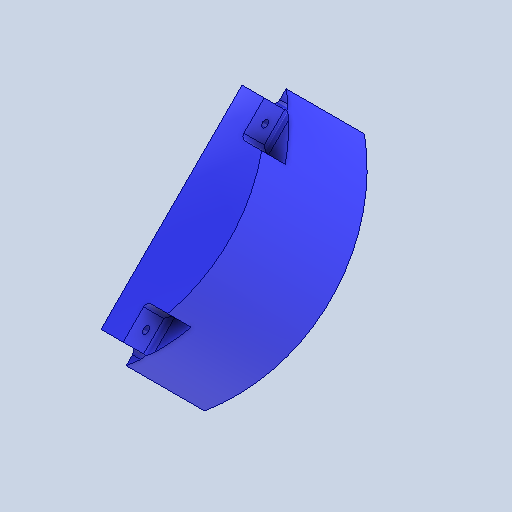
# Autodesk Inventor part: base_weel-v2-3DP-1
Saved by Autodesk Inventor 2025.2 (Build 292293000, 293)
## iProperties
Created: 2025-04-01
Part Number: base_weel-v2-3DP-1
Material: ABS プラスチック
Document SubType Name: Modeling
Designer: haruy
Density: 1.06 g/cm^3
Appearance: 青 - 壁塗料 - 光沢
Author: haruy
Autodesk Inventor part; units mm, degrees
ref_plane "YZ Plane" through (0, 0, 0) normal (1, 0, 0) x (0, 1, 0)
ref_plane "XZ Plane" through (0, 0, 0) normal (0, 1, 0) x (-1, 0, 0)
ref_plane "XY Plane" through (0, 0, 0) normal (0, 0, 1) x (1, 0, 0)
derived "base_weel-v2-Sketch-Base.ipt"
sketch "スケッチ1" plane through (0, 0, 0) normal (1, 0, 0) x (0, 1, 0)
  line L0 (-315, 315) -> (315, 315)
  line L1 (315, 315) -> (315, -315)
  line L2 (315, -315) -> (-315, -315)
  line L3 (-315, -315) -> (-315, 315)
  line L4 (-315, 315) -> (315, -315) construction
  line L5 (315, 315) -> (-315, -315) construction
  line L6 (-295, 218) -> (-295, -202)
  line L7 (-295, -202) -> (-315, -202)
  line L8 (-315, -202) -> (-315, 210)
  line L9 (242, 315) -> (-242, 315)
  line L10 (-242, 315) -> (-242, 295)
  line L11 (-242, 295) -> (242, 295)
  line L12 (242, 295) -> (242, 315)
  line L13 (-295, 218) -> (-295, 315)
  line L14 (0, 0) -> (-956.597305, 0)
  circle A0 centre (0, 0) radius 400
  line L15 (-330, 25) -> (-380, 25)
  line L16 (-380, 25) -> (-380, -25)
  line L17 (-380, -25) -> (-330, -25)
  line L18 (-330, -25) -> (-330, 25)
  line L19 (0, 0) -> (0, -630.91786)
  line L20 (-315, 40) -> (-395, 40)
  line L21 (-395, 40) -> (-395, 30)
  line L22 (-395, 30) -> (-315, 30)
  line L23 (-315, 30) -> (-315, 40)
  line L24 (-395, 30) -> (-385, 30)
  line L25 (-385, 30) -> (-385, 0)
  line L26 (-385, 0) -> (-395, 0)
  line L27 (-395, 0) -> (-395, 30)
  line L28 (295, 202) -> (315, 202)
  line L29 (315, 202) -> (315, -202)
  line L30 (315, -202) -> (295, -202)
  line L31 (295, -202) -> (295, 202)
  line L32 (-222.218254, -315) -> (242, -315)
  line L33 (242, -315) -> (242, -295)
  line L34 (242, -295) -> (-242, -295)
  line L35 (315, 315) -> (0, 0)
  line L36 (315, 125) -> (315, 145)
  circle A1 centre (548.476864, 0) radius 122.5
  circle A2 centre (179.690493, 0) radius 600
  circle A3 centre (548.476864, 0) radius 200
  circle A4 centre (0, 0) radius 10
  arc A5 (0, 150) -> (0, -150) centre (0, 0) ccw
  arc A6 (0, 140) -> (0, -140) centre (0, 0) ccw
  line L37 (-146.327154, 32.990361) -> (-136.572011, 30.791004)
  line L38 (-137.581214, 37.681687) -> (-140.440379, 25)
  line L39 (-140.440379, 25) -> (-145.317951, 26.099679)
  line L40 (-145.317951, 26.099679) -> (-142.458786, 38.781365)
  line L41 (-142.458786, 38.781365) -> (-137.581214, 37.681687)
  arc A7 (-29.130183, 142.04377) -> (-29.130183, -142.04377) centre (0, 0) ccw
  circle A8 centre (-151.490382, 39.279944) radius 6.5
  circle A9 centre (-129.040116, 34.218393) radius 6.5 construction
  circle A10 centre (-129.040116, 34.218393) radius 1.5 construction
  circle A11 centre (-151.490382, 39.279944) radius 1.5
  line L42 (-30.166794, 22.5) -> (-174.136226, 22.5)
  line L43 (-174.136226, 22.5) -> (-174.136226, 7.5)
  line L44 (-174.136226, 7.5) -> (-30.166794, 7.5)
  line L45 (-30.166794, 7.5) -> (-30.166794, 22.5)
  circle A12 centre (-129.040116, -34.218393) radius 6.5 construction
  circle A13 centre (-129.040116, -34.218393) radius 1.5 construction
  line L46 (-142.458786, -38.781365) -> (-137.581214, -37.681687)
  line L47 (-145.317951, -26.099679) -> (-142.458786, -38.781365)
  line L48 (-137.581214, -37.681687) -> (-140.440379, -25)
  line L49 (-140.440379, -25) -> (-145.317951, -26.099679)
  circle A14 centre (-151.490382, -39.279944) radius 6.5
  circle A15 centre (-151.490382, -39.279944) radius 1.5
  line L50 (-146.327154, -32.990361) -> (-136.572011, -30.791004)
  line L51 (-30.166794, -22.5) -> (-174.136226, -22.5)
  line L52 (-174.136226, -7.5) -> (-30.166794, -7.5)
  line L53 (-30.166794, -7.5) -> (-30.166794, -22.5)
  line L54 (-174.136226, -22.5) -> (-174.136226, -7.5)
  line L55 (-151.490382, 39.279944) -> (-129.040116, 34.218393) construction
  line L56 (-129.040116, 34.218393) -> (-129.589956, 31.779607) construction
  line L57 (-129.589956, 31.779607) -> (-152.040222, 36.841158) construction
  line L58 (-152.040222, 36.841158) -> (-151.490382, 39.279944) construction
  line L59 (-129.040116, 34.218393) -> (-151.490382, 39.279944) construction
  line L60 (-151.490382, 39.279944) -> (-150.940543, 41.71873) construction
  line L61 (-150.940543, 41.71873) -> (-128.490277, 36.657179) construction
  line L62 (-128.490277, 36.657179) -> (-129.040116, 34.218393) construction
  line L63 (-128.490277, 36.657179) -> (-129.589956, 31.779607) construction
  line L64 (-129.589956, 31.779607) -> (-117.883783, 29.140378) construction
  line L65 (-117.883783, 29.140378) -> (-116.784104, 34.01795) construction
  line L66 (-116.784104, 34.01795) -> (-128.490277, 36.657179) construction
  line L67 (-150.940543, 41.71873) -> (-152.040222, 36.841158) construction
  line L68 (-152.040222, 36.841158) -> (-163.746394, 39.480387) construction
  line L69 (-163.746394, 39.480387) -> (-162.646715, 44.357959) construction
  line L70 (-162.646715, 44.357959) -> (-150.940543, 41.71873) construction
  line L71 (-155.268276, 45.257195) -> (-128.941244, 39.321603)
  line L72 (-128.941244, 39.321603) -> (-132.24028, 24.688887)
  line L73 (-132.24028, 24.688887) -> (-158.567312, 30.624479)
  line L74 (-158.567312, 30.624479) -> (-155.268276, 45.257195)
  line L75 (-128.941244, -39.321603) -> (-132.24028, -24.688887)
  line L76 (-155.268276, -45.257195) -> (-128.941244, -39.321603)
  line L77 (-132.24028, -24.688887) -> (-158.567312, -30.624479)
  line L78 (-158.567312, -30.624479) -> (-155.268276, -45.257195)
  arc A16 (-132.24028, 24.688887) -> (-132.24028, -24.688887) centre (0, 0) ccw
  arc A17 (-158.567312, 30.624479) -> (-158.567312, -30.624479) centre (0, 0) ccw
  circle A18 centre (-152.5, 15) radius 1.25
  line L79 (-145, 0) -> (-145, 74.738194)
  circle A19 centre (-137.5, 15) radius 1.25
  circle A20 centre (-137.5, -15) radius 1.25
  circle A21 centre (-152.5, -15) radius 1.25
  line L80 (0, 0) -> (0, 140)
  line L81 (0, 0) -> (-47.88282, 131.556967)
  line L82 (0, 140) -> (0, 150)
  line L83 (-137.584562, 25.893789) -> (-134.285526, 40.526504)
  line L84 (-137.584562, -25.893789) -> (-134.285526, -40.526504)
  circle A22 centre (0, 0) radius 20
  line L85 (295, 45) -> (-295, 45)
  line L86 (-295, 45) -> (-295, 25)
  line L87 (-295, 25) -> (295, 25)
  line L88 (295, 25) -> (295, 45)
  line L89 (-40, 295) -> (-50, 295)
  line L90 (-50, 295) -> (-50, 45)
  line L91 (-50, 45) -> (-40, 45)
  line L92 (-40, 45) -> (-40, 295)
  line L93 (-50, -295) -> (-50, -45)
  line L94 (-40, -45) -> (-40, -295)
  line L95 (295, -45) -> (-295, -45)
  line L96 (-295, -25) -> (295, -25)
  line L97 (-40, 45) -> (-40, -45)
  line L98 (40, 45) -> (40, -45)
  circle A23 centre (20, 35) radius 1.5
  circle A24 centre (-20, 35) radius 1.5
  circle A25 centre (-20, -35) radius 1.5
  circle A26 centre (20, -35) radius 1.5
  circle A27 centre (-45, 125) radius 1.5
  circle A28 centre (-45, 125) radius 5
  circle A29 centre (-130, 35) radius 5
  circle A30 centre (-130, 35) radius 1.5
  line L99 (-40, 134.164079) -> (-40, 125)
  line L100 (-50, 125) -> (-50, 130.766968)
  line L101 (-137.749773, 25) -> (-127.580079, 30.624616)
  line L102 (-132.570736, 45) -> (-126.365969, 38.434213)
  line L103 (-40, -134.164079) -> (-40, -125)
  circle A31 centre (-45, -125) radius 5
  circle A32 centre (-45, -125) radius 1.5
  line L104 (-50, -125) -> (-50, -130.766968)
  line L105 (-132.570736, -45) -> (-126.365969, -38.434213)
  circle A33 centre (-130, -35) radius 5
  circle A34 centre (-130, -35) radius 1.5
  line L106 (-137.749773, -25) -> (-127.580079, -30.624616)
  line L107 (-242, -295) -> (-242, -315)
  line L108 (242, 315) -> (222, 315)
  line L109 (222, 315) -> (222, 295)
  line L110 (222, 295) -> (242, 295)
  line L111 (242, 295) -> (242, 315)
  line L112 (242, -315) -> (222, -315)
  line L113 (222, -315) -> (222, -295)
  line L114 (222, -295) -> (242, -295)
  line L115 (242, -295) -> (242, -315)
  line L116 (197, 295) -> (295, 197)
  line L117 (295, 197) -> (284.393398, 186.393398)
  line L118 (284.393398, 186.393398) -> (186.393398, 284.393398)
  line L119 (186.393398, 284.393398) -> (197, 295)
  line L120 (197, 295) -> (197, 315)
  line L121 (197.916739, 294.083261) -> (187.310137, 283.476659)
  line L122 (198.270292, 272.516504) -> (272.516504, 198.270292)
  line L123 (272.516504, 198.270292) -> (231.504311, 157.258099)
  line L124 (231.504311, 157.258099) -> (157.258099, 231.504311)
  line L125 (157.258099, 231.504311) -> (198.270292, 272.516504)
  line L126 (290.901281, 201.098719) -> (280.294679, 190.492118)
  line L127 (93.76241, 295) -> (295, 93.76241)
  line L128 (295, 93.76241) -> (284.393398, 83.155808)
  line L129 (284.393398, 83.155808) -> (83.155808, 284.393398)
  line L130 (214.180195, 277.819805) -> (203.573593, 267.213203)
  line L131 (277.819805, 214.180195) -> (267.213203, 203.573593)
  circle A35 centre (199.684506, 281.708892) radius 1.5
  circle A36 centre (213.826641, 267.566757) radius 1.6
  line L132 (186.393398, 284.393398) -> (175.786797, 295)
  circle A37 centre (187, 305) radius 1.5
  circle A38 centre (177, 305) radius 1.5
  line L133 (172, 315) -> (172, 295)
  line L134 (93.76241, 295) -> (93.76241, 295)
  line L135 (93.76241, 295) -> (93.76241, 315)
  line L136 (83.155808, 284.393398) -> (72.549207, 295)
  line L137 (68.76241, 315) -> (68.76241, 295)
  line L138 (284.393398, 186.393398) -> (295, 175.786797)
  line L139 (295, 197) -> (315, 197)
  line L140 (295, 93.76241) -> (295, 93.76241)
  line L141 (284.393398, 83.155808) -> (295, 72.549207)
  line L142 (-197, 295) -> (-197, 315)
  line L143 (-172, 315) -> (-172, 295)
  line L144 (-93.76241, 295) -> (-93.76241, 315)
  line L145 (-68.76241, 315) -> (-68.76241, 295)
  line L146 (-83.155808, 284.393398) -> (-72.549207, 295)
  line L147 (-93.76241, 295) -> (-295, 93.76241)
  line L148 (-83.155808, 284.393398) -> (-93.76241, 295)
  line L149 (-284.393398, 83.155808) -> (-83.155808, 284.393398)
  line L150 (-295, 93.76241) -> (-284.393398, 83.155808)
  line L151 (-284.393398, 83.155808) -> (-295, 72.549207)
  line L152 (-272.516504, 198.270292) -> (-231.504311, 157.258099)
  line L153 (-157.258099, 231.504311) -> (-198.270292, 272.516504)
  line L154 (-284.393398, 186.393398) -> (-186.393398, 284.393398)
  line L155 (-186.393398, 284.393398) -> (-175.786797, 295)
  line L156 (-197, 295) -> (-295, 197)
  line L157 (-197.916739, 294.083261) -> (-187.310137, 283.476659)
  line L158 (-214.180195, 277.819805) -> (-203.573593, 267.213203)
  line L159 (-290.901281, 201.098719) -> (-280.294679, 190.492118)
  line L160 (-284.393398, 186.393398) -> (-295, 175.786797)
  line L161 (-295, 197) -> (-315, 197)
  line L162 (-93.76241, -295) -> (-295, -93.76241)
  line L163 (-284.393398, -83.155808) -> (-83.155808, -284.393398)
  line L164 (-295, -93.76241) -> (-284.393398, -83.155808)
  line L165 (-197, -295) -> (-295, -197)
  line L166 (-284.393398, -186.393398) -> (-186.393398, -284.393398)
  line L167 (-290.901281, -201.098719) -> (-280.294679, -190.492118)
  line L168 (-214.180195, -277.819805) -> (-203.573593, -267.213203)
  line L169 (-197.916739, -294.083261) -> (-187.310137, -283.476659)
  line L170 (-83.155808, -284.393398) -> (-93.76241, -295)
  line L171 (284.393398, -83.155808) -> (83.155808, -284.393398)
  line L172 (83.155808, -284.393398) -> (93.76241, -295)
  line L173 (93.76241, -295) -> (295, -93.76241)
  line L174 (284.393398, -186.393398) -> (186.393398, -284.393398)
  line L175 (197.916739, -294.083261) -> (187.310137, -283.476659)
  line L176 (197, -295) -> (295, -197)
  line L177 (290.901281, -201.098719) -> (280.294679, -190.492118)
  line L178 (295, -93.76241) -> (284.393398, -83.155808)
  line L179 (242, 295) -> (222, 295)
  arc A39 (0, 86) -> (0, -86) centre (0, 0) ccw construction
  circle A40 centre (-90.866661, 48.5) radius 21
  circle A41 centre (0, 0) radius 124
  circle A42 centre (-90.866661, 48.5) radius 17
  arc A43 (40.495146, 75.869251) -> (0, 86) centre (0, 0) ccw construction
  line L180 (-40, 45) -> (-50, 45)
  line L181 (-50, 45) -> (-50, -45)
  line L182 (-50, -45) -> (-40, -45)
  line L183 (-40, -45) -> (-40, 45)
  line L184 (-40, 295) -> (-50, 295)
  line L185 (-50, 295) -> (-50, 315)
  line L186 (-50, 315) -> (-40, 315)
  line L187 (-40, 315) -> (-40, 295)
  line L188 (-40, -295) -> (-50, -295)
  line L189 (-50, -295) -> (-50, -315)
  line L190 (-50, -315) -> (-40, -315)
  line L191 (-40, -315) -> (-40, -295)
  line L192 (40, -315) -> (40, -295)
  line L193 (50, -295) -> (50, -315)
  line L194 (50, -295) -> (50, -45)
  line L195 (40, -45) -> (40, -295)
  line L196 (40, -45) -> (40, 45)
  line L197 (50, 45) -> (50, -45)
  line L198 (40, 45) -> (40, 295)
  line L199 (50, 295) -> (50, 45)
  line L200 (40, 315) -> (40, 295)
  line L201 (50, 295) -> (50, 315)
  line L202 (-40.409176, 123.019006) -> (-35, 135.554417)
  line L203 (-48.741703, 121.683426) -> (-55, 128.743932)
  line L204 (-40.409176, -123.019006) -> (-35, -135.554417)
  line L205 (-48.741703, -121.683426) -> (-55, -128.743932)
  arc A44 (40.495146, 75.869251) -> (-40.495146, -75.869251) centre (0, 0) ccw
  circle A45 centre (0, 0) radius 86 construction
  circle A46 centre (0, 0) radius 78.5
  circle A47 centre (-45, 58) radius 1.5
  circle A48 centre (-45, 58) radius 5
  circle A49 centre (45, 58) radius 5
  circle A50 centre (45, 58) radius 1.5
  line L206 (46.554886, 53.247913) -> (55, 56.01116)
  line L207 (40.325005, 56.226748) -> (35, 70.265568)
  line L208 (50, 60.516527) -> (50, 69.971423)
  arc A51 (50, 69.971423) -> (40.495146, 75.869251) centre (0, 0) ccw
  line L209 (-40.325005, 56.226748) -> (-35, 70.265568)
  line L210 (-46.554886, 53.247913) -> (-55, 56.01116)
  line L211 (-40.325005, -56.226748) -> (-35, -70.265568) construction
  circle A52 centre (-45, -58) radius 5
  line L212 (-46.554886, -53.247913) -> (-55, -56.01116)
  circle A53 centre (-45, -58) radius 1.5
  line L213 (-40, -67.54443) -> (-40, -76.131465)
  arc A54 (-40.525953, -75.852799) -> (-40, -76.131465) centre (0, 0) ccw
  line L214 (-40, -76.131465) -> (-40, -58)
  line L215 (222.665476, 269.334524) -> (212.058875, 258.727922)
  line L216 (269.334524, 222.665476) -> (258.727922, 212.058875)
  circle A55 centre (267.566757, 213.826641) radius 1.6
  circle A56 centre (281.708892, 199.684506) radius 1.5
  line L217 (294.083261, 197.916739) -> (283.476659, 187.310137)
  line L218 (315, 172) -> (295, 172)
  circle A57 centre (305, 177) radius 1.5
  circle A58 centre (305, 187) radius 1.5
  line L219 (295, 197) -> (315, 197)
  circle A59 centre (83.76241, 305) radius 1.5
  circle A60 centre (73.76241, 305) radius 1.5
  line L220 (197.916739, 294.083261) -> (94.679149, 294.083261)
  line L221 (187.310137, 283.476659) -> (84.072547, 283.476659)
  line L222 (94.679149, 294.083261) -> (84.072547, 283.476659)
  circle A61 centre (96.446916, 281.708892) radius 1.5
  circle A62 centre (110.589051, 267.566757) radius 1.5
  line L223 (119.427886, 269.334524) -> (108.821284, 258.727922)
  line L224 (295, 93.76241) -> (315, 93.76241)
  line L225 (315, 68.76241) -> (295, 68.76241)
  circle A63 centre (305, 73.76241) radius 1.5
  circle A64 centre (305, 83.76241) radius 1.5
  line L226 (294.083261, 94.679149) -> (283.476659, 84.072547)
  circle A65 centre (281.708892, 96.446916) radius 1.5
  circle A66 centre (267.566757, 110.589051) radius 1.5
  line L227 (269.334524, 119.427886) -> (258.727922, 108.821284)
  line L228 (-197, 295) -> (-197, 315)
  line L229 (-172, 315) -> (-172, 295)
  circle A67 centre (-177, 305) radius 1.5
  circle A68 centre (-187, 305) radius 1.5
  line L230 (-197.916739, 294.083261) -> (-187.310137, 283.476659)
  circle A69 centre (-199.684506, 281.708892) radius 1.5
  line L231 (-214.180195, 277.819805) -> (-203.573593, 267.213203)
  circle A70 centre (-213.826641, 267.566757) radius 1.6
  line L232 (-222.665476, 269.334524) -> (-212.058875, 258.727922)
  circle A71 centre (-267.566757, 213.826641) radius 1.6
  line L233 (-269.334524, 222.665476) -> (-258.727922, 212.058875)
  circle A72 centre (-281.708892, 199.684506) radius 1.5
  line L234 (-294.083261, 197.916739) -> (-283.476659, 187.310137)
  line L235 (-295, 197) -> (-315, 197)
  circle A73 centre (-305, 187) radius 1.5
  circle A74 centre (-305, 177) radius 1.5
  line L236 (-315, 172) -> (-295, 172)
  line L237 (-295, 93.76241) -> (-315, 93.76241)
  line L238 (-315, 68.76241) -> (-295, 68.76241)
  circle A75 centre (-305, 73.76241) radius 1.5
  circle A76 centre (-305, 83.76241) radius 1.5
  line L239 (-294.083261, 94.679149) -> (-283.476659, 84.072547)
  circle A77 centre (-281.708892, 96.446916) radius 1.5
  circle A78 centre (-267.566757, 110.589051) radius 1.5
  line L240 (-269.334524, 119.427886) -> (-258.727922, 108.821284)
  line L241 (-119.427886, 269.334524) -> (-108.821284, 258.727922)
  circle A79 centre (-110.589051, 267.566757) radius 1.5
  circle A80 centre (-96.446916, 281.708892) radius 1.5
  line L242 (-94.679149, 294.083261) -> (-84.072547, 283.476659)
  line L243 (-93.76241, 295) -> (-93.76241, 315)
  line L244 (-68.76241, 315) -> (-68.76241, 295)
  circle A81 centre (-73.76241, 305) radius 1.5
  circle A82 centre (-83.76241, 305) radius 1.5
  line L245 (-295, -197) -> (-315, -197)
  circle A83 centre (-305, -187) radius 1.5
  circle A84 centre (-305, -177) radius 1.5
  line L246 (-315, -172) -> (-295, -172)
  line L247 (-294.083261, -197.916739) -> (-283.476659, -187.310137)
  circle A85 centre (-281.708892, -199.684506) radius 1.5
  circle A86 centre (-267.566757, -213.826641) radius 1.6
  line L248 (-269.334524, -222.665476) -> (-258.727922, -212.058875)
  line L249 (-222.665476, -269.334524) -> (-212.058875, -258.727922)
  circle A87 centre (-213.826641, -267.566757) radius 1.6
  circle A88 centre (-199.684506, -281.708892) radius 1.5
  line L250 (-197.916739, -294.083261) -> (-187.310137, -283.476659)
  line L251 (-197, -295) -> (-197, -315)
  circle A89 centre (-187, -305) radius 1.5
  circle A90 centre (-177, -305) radius 1.5
  line L252 (-172, -315) -> (-172, -295)
  line L253 (-295, -93.76241) -> (-315, -93.76241)
  circle A91 centre (-305, -83.76241) radius 1.5
  circle A92 centre (-305, -73.76241) radius 1.5
  line L254 (-315, -68.76241) -> (-295, -68.76241)
  line L255 (-294.083261, -94.679149) -> (-283.476659, -84.072547)
  circle A93 centre (-281.708892, -96.446916) radius 1.5
  circle A94 centre (-267.566757, -110.589051) radius 1.5
  line L256 (-269.334524, -119.427886) -> (-258.727922, -108.821284)
  line L257 (-119.427886, -269.334524) -> (-108.821284, -258.727922)
  circle A95 centre (-110.589051, -267.566757) radius 1.5
  circle A96 centre (-96.446916, -281.708892) radius 1.5
  line L258 (-94.679149, -294.083261) -> (-84.072547, -283.476659)
  line L259 (-93.76241, -295) -> (-93.76241, -315)
  circle A97 centre (-83.76241, -305) radius 1.5
  circle A98 centre (-73.76241, -305) radius 1.5
  line L260 (-68.76241, -315) -> (-68.76241, -295)
  line L261 (68.76241, -315) -> (68.76241, -295)
  circle A99 centre (73.76241, -305) radius 1.5
  circle A100 centre (83.76241, -305) radius 1.5
  line L262 (93.76241, -295) -> (93.76241, -315)
  line L263 (94.679149, -294.083261) -> (84.072547, -283.476659)
  circle A101 centre (96.446916, -281.708892) radius 1.5
  circle A102 centre (110.589051, -267.566757) radius 1.5
  line L264 (119.427886, -269.334524) -> (108.821284, -258.727922)
  line L265 (172, -315) -> (172, -295)
  circle A103 centre (177, -305) radius 1.5
  circle A104 centre (187, -305) radius 1.5
  line L266 (197, -295) -> (197, -315)
  line L267 (197.916739, -294.083261) -> (187.310137, -283.476659)
  circle A105 centre (199.684506, -281.708892) radius 1.5
  circle A106 centre (213.826641, -267.566757) radius 1.6
  line L268 (222.665476, -269.334524) -> (212.058875, -258.727922)
  line L269 (269.334524, -222.665476) -> (258.727922, -212.058875)
  circle A107 centre (267.566757, -213.826641) radius 1.6
  circle A108 centre (281.708892, -199.684506) radius 1.5
  line L270 (294.083261, -197.916739) -> (283.476659, -187.310137)
  line L271 (295, -197) -> (315, -197)
  circle A109 centre (305, -187) radius 1.5
  circle A110 centre (305, -177) radius 1.5
  line L272 (315, -172) -> (295, -172)
  line L273 (295, -93.76241) -> (315, -93.76241)
  circle A111 centre (305, -83.76241) radius 1.5
  circle A112 centre (305, -73.76241) radius 1.5
  line L274 (315, -68.76241) -> (295, -68.76241)
  line L275 (294.083261, -94.679149) -> (283.476659, -84.072547)
  circle A113 centre (281.708892, -96.446916) radius 1.5
  line L276 (269.334524, -119.427886) -> (258.727922, -108.821284)
  circle A114 centre (267.566757, -110.589051) radius 1.5
  line L277 (-295, 202) -> (-315, 202)
  line L278 (265, 45) -> (265, 25)
  circle A115 centre (275, 35) radius 1.5
  circle A116 centre (285, 35) radius 1.5
  circle A117 centre (305, 35) radius 1.5
  circle A118 centre (305, 25) radius 1.5
  line L279 (295, 25) -> (315, 25)
  line L280 (265, -45) -> (265, -25)
  circle A119 centre (275, -35) radius 1.5
  circle A120 centre (285, -35) radius 1.5
  circle A121 centre (305, -35) radius 1.5
  circle A122 centre (305, -25) radius 1.5
  circle A123 centre (-305, -25) radius 1.5
  circle A124 centre (-305, -35) radius 1.5
  circle A125 centre (-285, -35) radius 1.5
  circle A126 centre (-275, -35) radius 1.5
  line L281 (-265, -45) -> (-265, -25)
  line L282 (-265, 45) -> (-265, 25)
  circle A127 centre (-275, 35) radius 1.5
  circle A128 centre (-285, 35) radius 1.5
  circle A129 centre (-305, 35) radius 1.5
  circle A130 centre (-305, 25) radius 1.5
  circle A131 centre (48, 345) radius 44
  circle A132 centre (-50, 345) radius 44
  circle A133 centre (-50, 345) radius 15
  line L283 (295, 45) -> (315, 45)
  line L284 (295, 15) -> (315, 15)
  line L285 (-315, 45.5) -> (-390, 45.5)
  line L286 (-390, 45.5) -> (-390, 0)
  line L287 (-390, 0) -> (-315, 0)
  line L288 (-315, 0) -> (-315, 45.5)
  circle A134 centre (-305, 48) radius 1.5
  circle A135 centre (-305, -48) radius 1.5
  line L289 (114.787843, 210) -> (54.787843, 210)
  line L290 (54.787843, 210) -> (54.787843, 270)
  line L291 (54.787843, 270) -> (114.787843, 270)
  line L292 (114.787843, 270) -> (114.787843, 210)
  line L293 (34.787843, 210) -> (-25.212157, 210)
  line L294 (-25.212157, 210) -> (-25.212157, 270)
  line L295 (-25.212157, 270) -> (34.787843, 270)
  line L296 (34.787843, 270) -> (34.787843, 210)
  line L297 (-45.212157, 250) -> (-115.212157, 250)
  line L298 (-115.212157, 250) -> (-115.212157, 266)
  line L299 (-115.212157, 266) -> (-45.212157, 266)
  line L300 (-45.212157, 266) -> (-45.212157, 250)
  line L301 (-50.212157, 214) -> (-110.212157, 214)
  line L302 (-110.212157, 214) -> (-110.212157, 230)
  line L303 (-110.212157, 230) -> (-50.212157, 230)
  line L304 (-50.212157, 230) -> (-50.212157, 214)
  circle A136 centre (0, 0) radius 175.5
  line L305 (-185, -89) -> (-302, -89)
  line L306 (-302, -89) -> (-302, 89)
  line L307 (-302, 89) -> (-185, 89)
  line L308 (-185, 89) -> (-185, -89)
  line L309 (287, -17.787843) -> (205, -17.787843)
  line L310 (205, -17.787843) -> (205, 79.212157)
  line L311 (205, 79.212157) -> (287, 79.212157)
  line L312 (287, 79.212157) -> (287, -17.787843)
  line L313 (284.5, -114.787843) -> (207.5, -114.787843)
  line L314 (207.5, -114.787843) -> (207.5, -37.787843)
  line L315 (207.5, -37.787843) -> (284.5, -37.787843)
  line L316 (284.5, -37.787843) -> (284.5, -114.787843)
  line L317 (281, 99.212157) -> (211, 99.212157)
  line L318 (211, 99.212157) -> (211, 115.212157)
  line L319 (211, 115.212157) -> (281, 115.212157)
  line L320 (281, 115.212157) -> (281, 99.212157)
  line L321 (137.712157, 315) -> (-137.712157, 315)
  line L322 (-137.712157, 315) -> (-137.712157, 185)
  line L323 (-137.712157, 185) -> (137.712157, 185)
  line L324 (137.712157, 185) -> (137.712157, 315)
  line L325 (315, -137.712157) -> (185, -137.712157)
  line L326 (185, -137.712157) -> (185, 137.712157)
  line L327 (185, 137.712157) -> (315, 137.712157)
  line L328 (315, 137.712157) -> (315, -137.712157)
  line L329 (258.778175, 137.712157) -> (278.778175, 137.712157)
  line L330 (278.778175, 137.712157) -> (278.778175, 127.712157)
  line L331 (278.778175, 127.712157) -> (258.778175, 127.712157)
  line L332 (258.778175, 127.712157) -> (258.778175, 137.712157)
  circle A137 centre (268.778175, 132.712157) radius 1.5
  line L333 (278.778175, 137.712157) -> (231.198146, 137.712157)
  line L334 (231.198146, 137.712157) -> (231.198146, 147.712157)
  line L335 (231.198146, 147.712157) -> (278.778175, 147.712157)
  line L336 (278.778175, 147.712157) -> (278.778175, 137.712157)
  line L337 (255.192388, 112.356818) -> (233.979185, 133.570022)
  line L338 (233.979185, 133.570022) -> (230.443651, 130.034488)
  line L339 (230.443651, 130.034488) -> (251.656854, 108.821284)
  line L340 (251.656854, 108.821284) -> (255.192388, 112.356818)
  line L341 (288.77996, 89.375848) -> (114.124585, 264.031223)
  line L342 (269.334524, 126.498954) -> (265.79899, 122.96342)
  line L343 (248.12132, 147.712157) -> (269.334524, 126.498954)
  line L344 (244.585786, 144.176624) -> (248.12132, 147.712157)
  circle A138 centre (268.778175, 132.712157) radius 4
  line L345 (233.979185, 133.570022) -> (244.585786, 144.176624)
  line L346 (-330, 143.5) -> (-340, 143.5)
  line L347 (-340, 143.5) -> (-340, -143.5)
  line L348 (-340, -143.5) -> (-330, -143.5)
  line L349 (-330, -143.5) -> (-330, 143.5)
  line L350 (-315, 119) -> (-295, 119)
  line L351 (-295, 119) -> (-295, 104)
  line L352 (-295, 104) -> (-315, 104)
  line L353 (-315, 104) -> (-315, 119)
  line L354 (-315, 153.5) -> (-325, 153.5)
  line L355 (-325, 153.5) -> (-325, 0)
  line L356 (-325, 0) -> (-315, 0)
  line L357 (-315, 0) -> (-315, 153.5)
  line L358 (-340, 133.5) -> (-345, 133.5)
  line L359 (-345, 133.5) -> (-345, 143.5)
  line L360 (-345, 143.5) -> (-340, 143.5)
  line L361 (-340, 143.5) -> (-340, 133.5)
  line L362 (-330, 133.5) -> (-325, 133.5)
  line L363 (-325, 133.5) -> (-325, 143.5)
  line L364 (-325, 143.5) -> (-330, 143.5)
  line L365 (-330, 143.5) -> (-330, 133.5)
  line L366 (-325, 153.5) -> (-345, 153.5)
  line L367 (-345, 153.5) -> (-345, 143.5)
  line L368 (-345, 143.5) -> (-325, 143.5)
  line L369 (-325, 143.5) -> (-325, 153.5)
  line L370 (-295, 104) -> (-345, 104)
  line L371 (-345, 104) -> (-345, 98)
  line L372 (-345, 98) -> (-295, 98)
  line L373 (-295, 98) -> (-295, 104)
  line L374 (185, -25) -> (180, -25)
  line L375 (180, -25) -> (180, -15)
  line L376 (180, -15) -> (185, -15)
  line L377 (185, -15) -> (185, -25)
  line L378 (185, -25) -> (195, -25)
  line L379 (195, -25) -> (195, -15)
  line L380 (195, -15) -> (185, -15)
  line L381 (185, -15) -> (185, -25)
  line L382 (40, 180) -> (30, 180)
  line L383 (30, 180) -> (30, 195)
  line L384 (30, 195) -> (40, 195)
  line L385 (40, 195) -> (40, 180)
  circle A139 centre (-132.712157, 268.778175) radius 1.5
  circle A140 centre (132.712157, 268.778175) radius 1.5
  line L386 (-243.5, 89) -> (-243.5, -89)
  circle A141 centre (-214, 35) radius 1.5
  circle A142 centre (-214, -35) radius 1.5
  line L387 (-214, 89) -> (-214, -89)
  line L388 (-246, 89) -> (-246, -89)
  circle A143 centre (-254.5, 35) radius 4
  circle A144 centre (-254.5, -35) radius 4
  circle A145 centre (0, 0) radius 100
  circle A146 centre (-134.167143, -14.972565) radius 5
  circle A147 centre (-134.167143, -14.972565) radius 1.25
  circle A148 centre (-134.907376, -5) radius 5
  circle A149 centre (-134.907376, -5) radius 1.25
  line L389 (252.010408, 177.764196) -> (177.764196, 252.010408)
  point P0 (-141.449582, 31.890683)
  point P1 (-129.040116, 34.218393)
  point P2 (-150, 0)
  point P3 (-242, 305)
  point P4 (-295, 93.76241)
  point P5 (-161.497527, 0)
  point P6 (305, 25)
  point P7 (295, 35)
extrude "押し出し1" add sketch "スケッチ1" along normal blind 10 contours L116 L216 L118 L35 | L35 L118 L215 L116 | L215 L118 L130 L116 | L116 L131 L118 L216
sketch "スケッチ2" plane through (10, 267.213203, 203.573593) normal (0, -0.7071068, -0.7071068) x (-1, 0, 0)
  circle A0 centre (56.5, -45) radius 52.5
  line L0 (10, -90) -> (10, 0)
  line L1 (0, 0) -> (0, -90)
  line L2 (0, -45) -> (10, -45)
  circle A1 centre (56.5, -45) radius 62.5
  circle A2 centre (56.5, -45) radius 72.5
  line L3 (-16, -75) -> (-6, -75)
  line L4 (-6, -75) -> (-6, -15)
  line L5 (-6, -15) -> (-16, -15)
  line L6 (-16, -15) -> (-16, -75)
  line L7 (5, -96.029403) -> (5, -80.411862)
  line L8 (10, -45) -> (10, -49.047142)
  line L9 (-9.501894, -75) -> (0, -75)
  line L10 (-9.501894, -15) -> (0, -15)
  line L11 (-16, -45) -> (-6, -45)
  line L12 (5, 6.029403) -> (5, -9.588138)
  point P0 (5, -9.588138)
  point P1 (5, 6.029403)
  dimension "d3" = 105
  dimension "d4" = 46.5
  dimension "d5" = 0
  dimension "d6" = 10
  dimension "d7" = 10
  dimension "d8" = 10
  dimension "d9" = 60
  dimension "d10" = 30
  dimension "d11" = 5
  constraints: 22 end point, 7 point on line, 3 midpoint, 3 parallel, 3 point on circle, 2 centre point, 2 perpendicular, 2 symmetric about line, 1 horizontal, 1 tangent, 3 other
  measures "d3" diameter of A0
  measures "d4" distance from line of A0.centre L0
  measures "d5" distance from line of A0.centre L2
  measures "d8" distance of L5.end L4.end
  measures "d9" distance between parallel lines of L3 L5
  measures "d10" distance between parallel lines of L2 L3
  measures "d11" distance between parallel lines of L7 L0
extrude "押し出し2" add sketch "スケッチ2" along normal blind 50 contours A1 L1 L10 L5 A2 L12 | L7 A2 L3 L9 L1 A1 | A1 L4 L10 L1 | L1 L9 L4 A1 | L11 A2 L5 L4 | L4 L3 A2 L11
extrude "押し出し3" add sketch "スケッチ2" against normal blind 15 contours L1 A1 | A1 L4 L10 L1 | L1 L9 L4 A1 | L11 A2 L5 L4 | L4 L3 A2 L11
fillet "フィレット1" radius 2 11 edges at (10, 261.9099, 208.8769) (10, 261.9099, 219.4835) (10, 208.8769, 261.9099) (10, 219.4835, 261.9099) (7.5, 267.2132, 203.5736) (7.5, 203.5736, 267.2132) (5, 206.9635, 263.8233) (7.6746, 257.4316, 213.3552) (7.6746, 213.3552, 257.4316) (16, 235.3934, 235.3934) (5, 263.8233, 206.9635)
